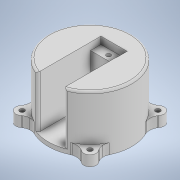
# Autodesk Inventor part: base1
Saved by Autodesk Inventor 2020.2 (Build 242310000, 310)
## iProperties
Created: 2026-05-19
Part Number: base1
Material: Generic
Document SubType Name: Modeling
Designer: explorer
Density: 1 g/cm^3
Appearance: Default
Author: explorer
Autodesk Inventor part; units mm, degrees
ref_plane "YZ Plane" through (0, 0, 0) normal (1, 0, 0) x (0, 1, 0)
ref_plane "XZ Plane" through (0, 0, 0) normal (0, 1, 0) x (-1, 0, 0)
ref_plane "XY Plane" through (0, 0, 0) normal (0, 0, 1) x (1, 0, 0)
sketch "Sketch2" plane through (0, 0, 0) normal (0, 1, 0) x (-1, 0, 0)
  circle A0 centre (0, 0) radius 20
  line L0 (6.25, -6.5) -> (-6.25, -6.5)
  line L1 (-6.25, -6.5) -> (-6.25, 22.6664)
  line L2 (-6.25, 22.6664) -> (6.25, 22.6664)
  line L3 (6.25, 22.6664) -> (6.25, -6.5)
  line L4 (0, -28.5333) -> (0, 31.1997) projected
  line L5 (28, 0) -> (-28, 0) projected
  point P0 (0, -6.5)
  point P1 (6.25, 18.9984)
  point P2 (-6.25, 18.9984)
  dimension "d5" = 40
  dimension "d6" = 6.5
  dimension "d7" = 12.5
  constraints: 8 end point, 2 parallel, 1 centre point, 1 coincident, 1 horizontal, 1 midpoint, 1 perpendicular, 1 point on line
  measures "d5" diameter of A0
  measures "d6" distance from line of L0 point (0, 0)
  measures "d7" distance of L0.start L0.end
extrude "Extrusion1" add sketch "Sketch2" along normal blind 25 contours L5 L3 A0 | A0 L4 L0 L3 L5 | A0 L5 L1 L0 L4 | A0 L1 L5
sketch "Sketch3" plane through (-6.25, 0, -6.5) normal (0, 0, 1) x (1, 0, 0)
  line L0 (0, 25) -> (12.5, 25) projected
  line L1 (0, 25) -> (12.6412, 25)
  line L2 (12.6412, 25) -> (12.6412, 21.5)
  line L3 (12.6412, 21.5) -> (0, 21.5)
  line L4 (0, 21.5) -> (0, 25)
  point P0 (0, 0)
  dimension "d10" = 3.5
  constraints: 8 end point, 2 parallel, 1 horizontal, 1 perpendicular
  measures "d10" distance of L1.end L2.end
extrude "Extrusion2" cut sketch "Sketch3" against normal blind 5
sketch "Sketch4" plane through (-6.25, 0, -6.5) normal (0, 0, 1) x (1, 0, 0)
  line L0 (0, 25) -> (12.5, 25)
  line L1 (0, 25) -> (12.6412, 25)
  line L2 (12.6412, 25) -> (12.6412, 21.5)
  line L3 (12.6412, 21.5) -> (0, 21.5)
  line L4 (0, 21.5) -> (0, 25)
  line L5 (0, 0) -> (12.5, 0)
  line L6 (0, 0) -> (12.6412, 0)
  line L7 (12.6412, 0) -> (12.6412, 6.5)
  line L8 (12.6412, 6.5) -> (0, 6.5)
  line L9 (0, 6.5) -> (0, 0)
  point P0 (6.25, 0)
  point P1 (6.25, 0)
  dimension "d15" = 3.5
  dimension "d16" = 15
  dimension "d17" = 6.5
  constraints: 20 end point, 4 parallel, 2 horizontal, 2 perpendicular
  measures "d15" distance of L1.end L2.end
  measures "d16" distance between parallel lines of L8 L3
  measures "d17" distance of L6.end L7.end
extrude "Extrusion3" cut sketch "Sketch4" against normal up to surface contours L9 L8 L7 L6 L5 round surface about axis through (0, 0, 0) along (0, 1, 0) radius 20 far side no
sketch "Sketch5" plane through (-6.25, 21.5, -6.5) normal (0, 1, 0) x (1, 0, 0)
  line L0 (12.6412, 0) -> (12.6412, 12.4513) projected
  line L1 (0, 0) -> (0, 12.4984) projected
  line L2 (0, 0) -> (6.25, 0)
  line L3 (6.25, 0) -> (6.25, 2.4)
  line L4 (6.25, 2.4) -> (0, 2.4)
  line L5 (0, 2.4) -> (0, 0)
  line L6 (12.5, 0) -> (0, 0) projected
  circle A0 centre (6.25, 2.4) radius 1.05
  point P0 (6.25, -6.5)
  dimension "d20" = 2.4
  dimension "d21" = 2.1
  constraints: 8 end point, 2 parallel, 1 centre point, 1 coincident, 1 horizontal, 1 midpoint, 1 perpendicular
  measures "d20" distance from line of L2 L4.end
  measures "d21" diameter of A0
extrude "Extrusion4" cut sketch "Sketch5" against normal up to surface (15 mm away) contours A0 L3 L4 | L4 L3 A0
sketch "Sketch6" plane through (0, 0, 0) normal (0, -1, 0) x (1, 0, 0)
  circle A0 centre (0, 0) radius 20
  constraints: 1 centre point, 1 coincident
extrude "Extrusion5" add sketch "Sketch6" along normal blind 2
sketch "Sketch8" plane through (0, -2, 0) normal (0, -1, 0) x (1, 0, 0)
  circle A0 centre (0, 0) radius 20
  line L0 (0, 0) -> (16.2635, -16.2635) construction
  line L1 (0, 0) -> (23, 0) construction
  circle A1 centre (0, 0) radius 20 projected
  arc A2 (18.2722, -8.1317) -> (18.2445, -13.897) centre (23.5204, -11.0397) ccw
  arc A3 (13.9222, -18.2518) -> (7.717, -18.3848) centre (10.9296, -23.4523) ccw
  line L2 (14.1421, -18.3848) -> (7.717, -18.3848) construction
  line L3 (14.1421, -18.3848) -> (20.5673, -18.3848) construction
  circle A4 centre (16.2635, -16.2635) radius 1.15
  arc A5 (14.2602, -18.4966) -> (18.5073, -14.2721) centre (16.2635, -16.2635) ccw
  arc A6 (18.2445, -13.897) -> (18.5073, -14.2721) centre (20.0031, -12.9446) ccw
  arc A7 (14.2602, -18.4966) -> (13.9222, -18.2518) centre (12.9246, -19.9853) ccw
  arc A8 (18.4966, 14.2602) -> (14.2721, 18.5073) centre (16.2635, 16.2635) ccw
  arc A9 (8.1317, 18.2722) -> (13.897, 18.2445) centre (11.0397, 23.5204) ccw
  arc A10 (18.2518, 13.9222) -> (18.3848, 7.717) centre (23.4523, 10.9296) ccw
  circle A11 centre (16.2635, 16.2635) radius 1.15
  arc A12 (13.897, 18.2445) -> (14.2721, 18.5073) centre (12.9446, 20.0031) ccw
  arc A13 (18.4966, 14.2602) -> (18.2518, 13.9222) centre (19.9853, 12.9246) ccw
  arc A14 (-14.2602, 18.4966) -> (-18.5073, 14.2721) centre (-16.2635, 16.2635) ccw
  arc A15 (-18.2722, 8.1317) -> (-18.2445, 13.897) centre (-23.5204, 11.0397) ccw
  arc A16 (-13.9222, 18.2518) -> (-7.717, 18.3848) centre (-10.9296, 23.4523) ccw
  circle A17 centre (-16.2635, 16.2635) radius 1.15
  arc A18 (-18.2445, 13.897) -> (-18.5073, 14.2721) centre (-20.0031, 12.9446) ccw
  arc A19 (-14.2602, 18.4966) -> (-13.9222, 18.2518) centre (-12.9246, 19.9853) ccw
  arc A20 (-18.4966, -14.2602) -> (-14.2721, -18.5073) centre (-16.2635, -16.2635) ccw
  arc A21 (-8.1317, -18.2722) -> (-13.897, -18.2445) centre (-11.0397, -23.5204) ccw
  arc A22 (-18.2518, -13.9222) -> (-18.3848, -7.717) centre (-23.4523, -10.9296) ccw
  circle A23 centre (-16.2635, -16.2635) radius 1.15
  arc A24 (-13.897, -18.2445) -> (-14.2721, -18.5073) centre (-12.9446, -20.0031) ccw
  arc A25 (-18.4966, -14.2602) -> (-18.2518, -13.9222) centre (-19.9853, -12.9246) ccw
  point P0 (17.9302, -8.8605)
  point P1 (9.4105, -17.6477)
  point P2 (8.8605, 17.9302)
  point P3 (17.6477, 9.4105)
  point P4 (-17.9302, 8.8605)
  point P5 (-9.4105, 17.6477)
  point P6 (-8.8605, -17.9302)
  point P7 (-17.6477, -9.4105)
  dimension "d38" = 40
  dimension "d39" = 23
  dimension "d40" = 45
  dimension "d42" = 6
  dimension "d44" = 6
  dimension "d45" = 2.3
  dimension "d46" = 2
  dimension "d51" = 360
  constraints: 42 point on circle, 25 centre point, 8 end point, 5 coincident, 4 tangent, 2 equal length, 2 horizontal, 1 equal radius, 75 other
  measures "d38" diameter of A0
  measures "d39" distance of L0.start L0.end
  measures "d40" angle of L0 L1
  measures "d42" radius of A2
  measures "d44" radius of A3
  measures "d45" diameter of A4
  measures "d46" radius of A6
extrude "Extrusion7" add sketch "Sketch8" against normal blind 5 contours A2 A6 A5 A7 A3 A0 | A0 A9 A12 A8 A13 A10 | A21 A24 A20 A25 A22 A0 | A0 A15 A18 A14 A19 A16
fillet "Fillet1" radius 5 10 edges at (17.9302, 0.5, -8.8605) (17.6477, 1.5, 9.4105) (17.6477, -1, 9.4105) (8.8605, -1, 17.9302) (8.8605, 1.5, 17.9302) (-9.4105, 0.5, 17.6477) (-17.9302, 0.5, 8.8605) (-17.6477, 0.5, -9.4105) (-8.8605, 0.5, -17.9302) (9.4105, 0.5, -17.6477)
fillet "Fillet1" radius 1 7 edges at (6.3912, 3.25, -18.9513) (0.0744, 0, -19.9999) (-6.25, 3.25, -18.9984) (0.0744, 6.5, -19.9999) (-6.25, 12.5, 18.9984) (6.25, 12.5, 18.9984) (0, 25, -20)
body "Solid1"
